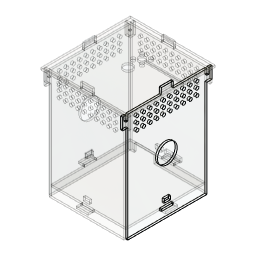
Cage_v8 (Autodesk Fusion 360 design; units mm, degrees)
Autodesk Fusion 360 part; units mm, degrees
(part 1 of 2)
sketch "Sketch1" plane through (0, 0, 0) normal (0, 0, 1) x (1, 0, 0)
  line L0 (-150, 3.175) -> (150, 3.175)
  line L1 (150, 3.175) -> (150, -3.175)
  line L2 (150, -3.175) -> (-150, -3.175)
  line L3 (-150, -3.175) -> (-150, 3.175)
  dimension "d1" = 300
  dimension "d2" = 150
  dimension "d3" = 6.35
  dimension "d4" = 3.175
  constraint horizontal L0
  constraint vertical L1
  constraint horizontal L2
  constraint vertical L3
  measures "d1" distance of L0.start L0.end
  measures "d2" distance of origin L3
  measures "d3" distance of L0.end L1.end
  measures "d4" distance of origin L0
extrude "Extrude1" add sketch "Sketch1" along normal blind 350 makes body 1
sketch "Sketch2" plane through (0, -3.175, 0) normal (0, -1, 0) x (1, 0, 0)
  line L0 (-150, 0) -> (150, 0)
  line L1 (150, 0) -> (150, 350)
  line L2 (150, 350) -> (-150, 350)
  line L3 (-150, 350) -> (-150, 0)
  line L4 (-120, 0) -> (120, 0)
  line L5 (120, 0) -> (120, 330.95)
  line L6 (120, 350) -> (-120, 350)
  line L7 (-120, 330.95) -> (-120, 0)
  line L8 (120, 350) -> (136.5, 350)
  line L9 (136.5, 350) -> (136.5, 311.9)
  line L10 (136.5, 311.9) -> (126.35, 311.9)
  line L11 (126.35, 311.9) -> (126.35, 330.95)
  line L12 (126.35, 330.95) -> (120, 330.95)
  line L13 (-120, 350) -> (-136.5, 350)
  line L14 (-136.5, 350) -> (-136.5, 311.9)
  line L15 (-136.5, 311.9) -> (-126.35, 311.9)
  line L16 (-126.35, 311.9) -> (-126.35, 330.95)
  line L17 (-126.35, 330.95) -> (-120, 330.95)
  dimension "d7" = 350
  dimension "d8" = 240
  dimension "d9" = 120
  dimension "d10" = 6.35
  dimension "d14" = 38.1
  dimension "d15" = 19.05
  dimension "d18" = 6.35
  dimension "d20" = 273
  dimension "d21" = 38.1
  dimension "d22" = 19.05
  constraint horizontal L4
  constraint vertical L5
  constraint horizontal L6
  constraint vertical L7
  constraint coincident L0 L4.start
  constraint coincident L2 L8.end
  constraint perpendicular L5 L8
  constraint perpendicular L2 L9
  constraint perpendicular L9 L10
  constraint perpendicular L10 L11
  constraint perpendicular L5 L12
  constraint coincident L2 L13.end
  constraint perpendicular L7 L13
  constraint perpendicular L13 L14
  constraint perpendicular L14 L15
  constraint perpendicular L15 L16
  constraint perpendicular L7 L17
  constraint equal L10 L15
  measures "d7" distance of L4.end L6.start
  measures "d8" distance of L4.start L4.end
  measures "d9" distance of origin L7
  measures "d10" distance of L11.end L5.end
  measures "d14" distance of L8.end L9.end
  measures "d15" distance of L8 L12
  measures "d18" distance of L16.end L7.start
  measures "d20" distance of L9 L14
  measures "d21" distance of L13.end L14.end
  measures "d22" distance of L13 L17
extrude "Extrude2" cut sketch "Sketch2" against normal blind 140 contours L0 L2 L3 L7 L14 L15 L16 L17 | L0 L1 L2 L5 L9 L10 L11 L12 bodies 1
sketch "Sketch3" plane through (0, 0, 350) normal (0, 0, 1) x (-1, 0, 0)
  line L0 (136.5, -3.175) -> (136.5, 3.175)
  line L1 (136.5, 3.175) -> (-136.5, 3.175)
  line L2 (-136.5, 3.175) -> (-136.5, -3.175)
  line L3 (-136.5, -3.175) -> (136.5, -3.175)
  line L4 (19.05, -3.175) -> (-19.05, -3.175)
  line L5 (-19.05, -3.175) -> (-19.05, 3.175)
  line L6 (-19.05, 3.175) -> (19.05, 3.175)
  line L7 (19.05, 3.175) -> (19.05, -3.175)
  dimension "d25" = 38.1
  dimension "d26" = 19.05
  constraint horizontal L4
  constraint vertical L5
  constraint horizontal L6
  constraint vertical L7
  constraint coincident L1 L5.end
  constraint coincident L3 L4.start
  measures "d25" distance of L4.start L4.end
  measures "d26" distance of origin L7
extrude "Extrude3" add sketch "Sketch3" along normal blind 20 contours L1 L3 L4 L5 L6 L7 bodies 1
sketch "Sketch4" plane through (0, -3.175, 0) normal (0, -1, 0) x (1, 0, 0)
  line L0 (-136.5, 350) -> (-136.5, 311.9)
  line L1 (-136.5, 311.9) -> (-126.35, 311.9)
  line L2 (-126.35, 311.9) -> (-126.35, 330.95)
  line L3 (-126.35, 330.95) -> (-120, 330.95)
  line L4 (-120, 330.95) -> (-120, 0)
  line L5 (-120, 0) -> (120, 0)
  line L6 (120, 0) -> (120, 330.95)
  line L7 (120, 330.95) -> (126.35, 330.95)
  line L8 (126.35, 330.95) -> (126.35, 311.9)
  line L9 (126.35, 311.9) -> (136.5, 311.9)
  line L10 (136.5, 311.9) -> (136.5, 350)
  line L11 (136.5, 350) -> (19.05, 350)
  line L12 (19.05, 350) -> (19.05, 370)
  line L13 (19.05, 370) -> (-19.05, 370)
  line L14 (-19.05, 370) -> (-19.05, 350)
  line L15 (-19.05, 350) -> (-136.5, 350)
  circle A0 centre (-90, 330) radius 5
  circle A1 centre (-70, 330) radius 5
  circle A2 centre (-50, 330) radius 5
  circle A3 centre (-30, 330) radius 5
  circle A4 centre (-10, 330) radius 5
  circle A5 centre (10, 330) radius 5
  circle A6 centre (30, 330) radius 5
  circle A7 centre (50, 330) radius 5
  circle A8 centre (70, 330) radius 5
  circle A9 centre (90, 330) radius 5
  circle A10 centre (-90, 310) radius 5
  circle A11 centre (-70, 310) radius 5
  circle A12 centre (-50, 310) radius 5
  circle A13 centre (-30, 310) radius 5
  circle A14 centre (-10, 310) radius 5
  circle A15 centre (10, 310) radius 5
  circle A16 centre (30, 310) radius 5
  circle A17 centre (50, 310) radius 5
  circle A18 centre (70, 310) radius 5
  circle A19 centre (90, 310) radius 5
  circle A20 centre (-90, 290) radius 5
  circle A21 centre (-70, 290) radius 5
  circle A22 centre (-50, 290) radius 5
  circle A23 centre (-30, 290) radius 5
  circle A24 centre (-10, 290) radius 5
  circle A25 centre (10, 290) radius 5
  circle A26 centre (30, 290) radius 5
  circle A27 centre (50, 290) radius 5
  circle A28 centre (70, 290) radius 5
  circle A29 centre (90, 290) radius 5
  dimension "d29" = 30
  dimension "d30" = 20
  dimension "d31" = 10
  dimension "d32" = 10
  dimension "d33" = 20
  dimension "d34" = 20
  dimension "d35" = 20
  dimension "d36" = 20
  dimension "d37" = 20
  dimension "d38" = 20
  dimension "d39" = 20
  dimension "d40" = 20
  dimension "d41" = 30
  dimension "d42" = 30
  dimension "d52" = 10
  dimension "d53" = 20
  dimension "d54" = 20
  dimension "d55" = 20
  dimension "d56" = 20
  dimension "d57" = 20
  dimension "d58" = 20
  dimension "d59" = 20
  dimension "d60" = 20
  dimension "d61" = 20
  dimension "d62" = 10
  dimension "d63" = 10
  constraint equal A7 A9
  constraint equal A6 A9
  constraint equal A5 A9
  constraint equal A4 A8
  constraint equal A3 A8
  constraint equal A2 A8
  constraint equal A1 A9
  constraint equal A0 A8
  constraint equal A18 A19
  constraint equal A17 A19
  constraint equal A16 A19
  constraint equal A15 A19
  constraint equal A14 A19
  constraint equal A13 A19
  constraint equal A12 A19
  constraint equal A11 A19
  constraint equal A10 A19
  measures "d29" distance of L6 A9.centre
  measures "d30" distance of A8.centre A9.centre
  measures "d31" diameter of A9
  measures "d32" diameter of A8
  measures "d33" distance of A7.centre A8.centre
  measures "d34" distance of A6.centre A7.centre
  measures "d35" distance of A5.centre A6.centre
  measures "d36" distance of A4.centre A5.centre
  measures "d37" distance of A3.centre A4.centre
  measures "d38" distance of A2.centre A3.centre
  measures "d39" distance of A1.centre A2.centre
  measures "d40" distance of A0.centre A1.centre
  measures "d41" distance of L4 A10.centre
  measures "d42" distance of L6 A19.centre
  measures "d52" diameter of A19
  measures "d53" distance of A18.centre A19.centre
  measures "d54" distance of A17.centre A18.centre
  measures "d55" distance of A16.centre A17.centre
  measures "d56" distance of A15.centre A16.centre
  measures "d57" distance of A14.centre A15.centre
  measures "d58" distance of A13.centre A14.centre
  measures "d59" distance of A12.centre A13.centre
  measures "d60" distance of A11.centre A12.centre
  measures "d61" distance of A10.centre A11.centre
  measures "d62" diameter of A20
  measures "d63" diameter of A21
extrude "Extrude4" cut sketch "Sketch4" against normal blind 35 contours A0 | A1 | A2 | A3 | A4 | A5 | A6 | A7 | A8 | A9 | A10 | A11 | A12 | A13 | A14 | A15 | A16 | A17 | A18 | A19 | A20 | A21 | A22 | A23 | A24 | A25 | A26 | A27 | A28 | A29 bodies 1
ref_plane "WorkPlane1" through (120, 0, 0) normal (1, 0, 0) x (0, 1, 0) in component "Right wall"
sketch "Sketch1 (2)" plane through (120, 0, 0) normal (1, 0, 0) x (0, 1, 0) in component "Right wall"
  line L0 (3.175, 0) -> (257.175, 0)
  line L1 (257.175, 0) -> (257.175, 350)
  line L2 (257.175, 350) -> (3.175, 350)
  line L3 (3.175, 350) -> (3.175, 0)
  dimension "d67" = 3.175
  dimension "d68" = 254
  dimension "d69" = 350
  constraint horizontal L0
  constraint vertical L1
  constraint horizontal L2
  constraint vertical L3
  measures "d67" distance of origin L0.start
  measures "d68" distance of L0.start L0.end
  measures "d69" distance of L0.end L1.end
extrude "Extrude1'" add sketch "Sketch1 (2)" along normal blind 6.35 separate body makes body 2 in component "Right wall"
sketch "Sketch2 (2)" plane through (0, 0, 350) normal (0, 0, 1) x (-1, 0, 0) in component "Right wall"
  line L0 (-120, -257.175) -> (-120, -3.175)
  line L1 (-120, -3.175) -> (-126.35, -3.175)
  line L2 (-126.35, -3.175) -> (-126.35, -257.175)
  line L3 (-126.35, -257.175) -> (-120, -257.175)
  line L4 (-126.35, -111.125) -> (-120, -111.125)
  line L5 (-120, -111.125) -> (-120, -149.225)
  line L6 (-120, -149.225) -> (-126.35, -149.225)
  line L7 (-126.35, -149.225) -> (-126.35, -111.125)
  dimension "d72" = 38.1
  dimension "d73" = 107.95
  constraint horizontal L4
  constraint vertical L5
  constraint horizontal L6
  constraint vertical L7
  constraint coincident L0 L5.end
  constraint coincident L2 L4.start
  measures "d72" distance of L4.end L5.end
  measures "d73" distance of L1 L4
extrude "Extrude2'" add sketch "Sketch2 (2)" along normal blind 20 contours L0 L2 L4 L5 L6 L7 bodies 2 in component "Right wall"
sketch "Sketch3 (2)" plane through (126.35, 0, 0) normal (1, 0, 0) x (0, 1, 0) in component "Right wall"
  line L0 (3.175, 350) -> (3.175, 0)
  line L1 (3.175, 0) -> (257.175, 0)
  line L2 (257.175, 0) -> (257.175, 350)
  line L3 (257.175, 350) -> (149.225, 350)
  line L4 (149.225, 350) -> (149.225, 370)
  line L5 (149.225, 370) -> (111.125, 370)
  line L6 (111.125, 370) -> (111.125, 350)
  line L7 (111.125, 350) -> (3.175, 350)
  circle A0 centre (33.875, 330) radius 5
  circle A1 centre (55.275, 330) radius 5
  circle A2 centre (76.675, 330) radius 5
  circle A3 centre (98.075, 330) radius 5
  circle A4 centre (119.475, 330) radius 5
  circle A5 centre (140.875, 330) radius 5
  circle A6 centre (162.275, 330) radius 5
  circle A7 centre (183.675, 330) radius 5
  circle A8 centre (205.075, 330) radius 5
  circle A9 centre (226.475, 330) radius 5
  circle A10 centre (33.875, 310) radius 5
  circle A11 centre (55.275, 310) radius 5
  circle A12 centre (76.675, 310) radius 5
  circle A13 centre (98.075, 310) radius 5
  circle A14 centre (119.475, 310) radius 5
  circle A15 centre (140.875, 310) radius 5
  circle A16 centre (162.275, 310) radius 5
  circle A17 centre (183.675, 310) radius 5
  circle A18 centre (205.075, 310) radius 5
  circle A19 centre (226.4722, 310.344) radius 5
  circle A20 centre (33.875, 290) radius 5
  circle A21 centre (55.275, 290) radius 5
  circle A22 centre (119.475, 290) radius 5
  circle A23 centre (140.875, 290) radius 5
  circle A24 centre (162.275, 290) radius 5
  circle A25 centre (98.075, 290) radius 5
  circle A26 centre (76.675, 290) radius 5
  circle A27 centre (183.675, 290) radius 5
  circle A28 centre (205.075, 290) radius 5
  circle A29 centre (226.475, 290) radius 5
  dimension "d76" = 20
  dimension "d77" = 10
  dimension "d78" = 30.7
  dimension "d79" = 21.4
  dimension "d80" = 21.4
  dimension "d81" = 21.4
  dimension "d82" = 21.4
  dimension "d85" = 21.4
  dimension "d86" = 21.4
  dimension "d87" = 21.4
  dimension "d88" = 21.4
  dimension "d90" = 20
  dimension "d91" = 10
  dimension "d92" = 30.7
  dimension "d93" = 21.4
  dimension "d94" = 21.4
  dimension "d95" = 21.4
  dimension "d96" = 21.4
  dimension "d99" = 21.4
  dimension "d100" = 21.4
  dimension "d101" = 21.4
  dimension "d102" = 21.4
  dimension "d103" = 21.4
  dimension "d104" = 21.4
  dimension "d105" = 10
  dimension "d106" = 21.4
  dimension "d107" = 21.4
  dimension "d108" = 21.4
  dimension "d109" = 21.4
  dimension "d110" = 21.4
  dimension "d111" = 21.4
  dimension "d112" = 21.4
  dimension "d113" = 21.4
  dimension "d114" = 21.4
  dimension "d211" = 20
  dimension "d212" = 30.7
  constraint equal A0 A1
  constraint equal A0 A2
  constraint equal A0 A3
  constraint equal A3 A4
  constraint equal A5 A6
  constraint equal A6 A7
  constraint equal A7 A8
  constraint equal A8 A9
  constraint collinear A0.centre A1.centre A2.centre
  constraint collinear A5.centre A6.centre A7.centre
  constraint collinear A7.centre A8.centre A9.centre
  constraint collinear A10.centre A11.centre A12.centre
  constraint equal A10 A11
  constraint equal A11 A12
  constraint equal A12 A13
  constraint equal A13 A14
  constraint equal A15 A16
  constraint equal A16 A17
  constraint equal A17 A18
  constraint equal A18 A19
  constraint equal A14 A15
  constraint equal A4 A5
  constraint collinear A26.centre A20.centre A21.centre
  constraint equal A20 A21
  constraint equal A21 A26
  constraint equal A25 A26
  constraint equal A22 A25
  constraint equal A23 A24
  constraint equal A24 A27
  constraint equal A27 A28
  constraint equal A28 A29
  constraint equal A22 A23
  measures "d76" distance of L7 A0.centre
  measures "d77" diameter of A0
  measures "d78" distance of L0 A0.centre
  measures "d79" distance of A0.centre A1.centre
  measures "d80" distance of A1.centre A2.centre
  measures "d81" distance of A2.centre A3.centre
  measures "d82" distance of A3.centre A4.centre
  measures "d85" distance of A5.centre A6.centre
  measures "d86" distance of A6.centre A7.centre
  measures "d87" distance of A7.centre A8.centre
  measures "d88" distance of A8.centre A9.centre
  measures "d90" vertical distance of A0.centre A10.centre
  measures "d91" diameter of A10
  measures "d92" distance of L0 A10.centre
  measures "d93" distance of A10.centre A11.centre
  measures "d94" distance of A11.centre A12.centre
  measures "d95" distance of A12.centre A13.centre
  measures "d96" distance of A13.centre A14.centre
  measures "d99" distance of A15.centre A16.centre
  measures "d100" distance of A16.centre A17.centre
  measures "d101" distance of A17.centre A18.centre
  measures "d102" distance of A18.centre A19.centre
  measures "d103" distance of A4.centre A5.centre
  measures "d104" distance of A14.centre A15.centre
  measures "d105" diameter of A20
  measures "d106" distance of A20.centre A21.centre
  measures "d107" distance of A26.centre A21.centre
  measures "d108" distance of A26.centre A25.centre
  measures "d109" distance of A25.centre A22.centre
  measures "d110" distance of A23.centre A24.centre
  measures "d111" distance of A27.centre A24.centre
  measures "d112" distance of A27.centre A28.centre
  measures "d113" distance of A29.centre A28.centre
  measures "d114" distance of A23.centre A22.centre
  measures "d211" vertical distance of A10.centre A20.centre
  measures "d212" distance of L2 A29.centre
extrude "Extrude3'" cut sketch "Sketch3 (2)" against normal blind 40 contours A0 | A1 | A2 | A3 | A4 | A5 | A6 | A7 | A8 | A9 | A10 | A11 | A12 | A13 | A14 | A15 | A16 | A17 | A18 | A19 | A20 | A21 | A22 | A23 | A24 | A25 | A26 | A27 | A28 | A29 bodies 2 in component "Right wall"
sketch "Sketch5" plane through (126.35, 0, 0) normal (1, 0, 0) x (0, 1, 0) in component "Right wall"
  circle A0 centre (183.675, 290) radius 5
  circle A1 centre (98.075, 290) radius 5
  circle A2 centre (33.875, 310) radius 5
  circle A3 centre (119.475, 310) radius 5
  circle A4 centre (205.075, 310) radius 5
  circle A5 centre (183.675, 330) radius 5
  circle A6 centre (98.075, 330) radius 5
  circle A7 centre (33.875, 330) radius 5
  circle A8 centre (119.475, 330) radius 5
  circle A9 centre (205.075, 330) radius 5
  circle A10 centre (183.675, 310) radius 5
  circle A11 centre (98.075, 310) radius 5
  circle A12 centre (33.875, 290) radius 5
  circle A13 centre (119.475, 290) radius 5
  circle A14 centre (205.075, 290) radius 5
  circle A15 centre (162.275, 290) radius 5
  circle A16 centre (76.675, 290) radius 5
  circle A17 centre (55.275, 310) radius 5
  circle A18 centre (162.275, 310) radius 5
  circle A19 centre (226.4722, 310.344) radius 5
  circle A20 centre (162.275, 330) radius 5
  circle A21 centre (76.675, 330) radius 5
  circle A22 centre (55.275, 330) radius 5
  circle A23 centre (140.875, 330) radius 5
  circle A24 centre (226.475, 330) radius 5
  circle A25 centre (140.875, 310) radius 5
  circle A26 centre (76.675, 310) radius 5
  circle A27 centre (55.275, 290) radius 5
  circle A28 centre (140.875, 290) radius 5
  circle A29 centre (226.475, 290) radius 5
  line L0 (3.175, 350) -> (3.175, 0)
  line L1 (3.175, 0) -> (257.175, 0)
  line L2 (257.175, 0) -> (257.175, 350)
  line L3 (257.175, 350) -> (149.225, 350)
  line L4 (149.225, 350) -> (149.225, 370)
  line L5 (149.225, 370) -> (111.125, 370)
  line L6 (111.125, 370) -> (111.125, 350)
  line L7 (111.125, 350) -> (3.175, 350)
  line L8 (3.175, 311.9) -> (-13.325, 311.9)
  line L9 (-3.175, 330.95) -> (3.175, 330.95)
  line L10 (3.175, 330.95) -> (3.175, 311.9)
  line L11 (-13.325, 350) -> (-3.175, 350)
  line L12 (-3.175, 350) -> (-3.175, 330.95)
  line L13 (257.175, 311.9) -> (273.675, 311.9)
  line L14 (273.675, 311.9) -> (273.675, 350)
  line L15 (273.675, 350) -> (263.525, 350)
  line L16 (263.525, 350) -> (263.525, 330.95)
  line L17 (263.525, 330.95) -> (257.175, 330.95)
  line L18 (-13.325, 350) -> (-13.325, 311.9)
  dimension "d119" = 19.05
  dimension "d124" = 6.35
  dimension "d127" = 6.35
  dimension "d128" = 10.15
  dimension "d130" = 19.05
  dimension "d131" = 19.05
  dimension "d132" = 19.05
  dimension "d133" = 19.05
  constraint horizontal L8
  constraint horizontal L9
  constraint vertical L10
  constraint coincident L0 L8.start
  constraint horizontal L11
  constraint vertical L12
  constraint coincident L2 L13.start
  constraint perpendicular L2 L13
  constraint perpendicular L13 L14
  constraint perpendicular L14 L15
  constraint perpendicular L15 L16
  constraint coincident L2 L17.end
  constraint perpendicular L2 L17
  constraint perpendicular L8 L18
  measures "d119" distance of L7 L9
  measures "d124" distance of L0 L12
  measures "d127" distance of L16.end L17.end
  measures "d128" distance of L14.end L15.end
  measures "d130" distance of L13 L17
  measures "d131" distance of L15.end L16.end
  measures "d132" distance of L9 L11
  measures "d133" distance of L8 L9
extrude "Extrude4'" add sketch "Sketch5" against normal blind 6.35 contours L0 L8 L9 L10 L11 L12 L18 | L2 L13 L14 L15 L16 L17 bodies 2 in component "Right wall"
sketch "Sketch5 (2)" plane through (0, -3.175, 0) normal (0, -1, 0) x (1, 0, 0)
  circle A0 centre (50, 290) radius 5
  circle A1 centre (-30, 290) radius 5
  circle A2 centre (-90, 310) radius 5
  circle A3 centre (-10, 310) radius 5
  circle A4 centre (70, 310) radius 5
  circle A5 centre (50, 330) radius 5
  circle A6 centre (-30, 330) radius 5
  circle A7 centre (-90, 330) radius 5
  circle A8 centre (-10, 330) radius 5
  circle A9 centre (70, 330) radius 5
  circle A10 centre (50, 310) radius 5
  circle A11 centre (-30, 310) radius 5
  circle A12 centre (-90, 290) radius 5
  circle A13 centre (-10, 290) radius 5
  circle A14 centre (70, 290) radius 5
  circle A15 centre (30, 290) radius 5
  circle A16 centre (-50, 290) radius 5
  circle A17 centre (-70, 310) radius 5
  circle A18 centre (10, 310) radius 5
  circle A19 centre (90, 310) radius 5
  circle A20 centre (30, 330) radius 5
  circle A21 centre (-50, 330) radius 5
  circle A22 centre (-70, 330) radius 5
  circle A23 centre (10, 330) radius 5
  circle A24 centre (90, 330) radius 5
  circle A25 centre (30, 310) radius 5
  circle A26 centre (-50, 310) radius 5
  circle A27 centre (-70, 290) radius 5
  circle A28 centre (10, 290) radius 5
  circle A29 centre (90, 290) radius 5
  line L0 (-136.5, 350) -> (-136.5, 311.9)
  line L1 (-136.5, 311.9) -> (-126.35, 311.9)
  line L2 (-126.35, 311.9) -> (-126.35, 330.95)
  line L3 (-126.35, 330.95) -> (-120, 330.95)
  line L4 (-120, 330.95) -> (-120, 0)
  line L5 (-120, 0) -> (120, 0)
  line L6 (120, 0) -> (120, 330.95)
  line L7 (120, 330.95) -> (126.35, 330.95)
  line L8 (126.35, 330.95) -> (126.35, 311.9)
  line L9 (126.35, 311.9) -> (136.5, 311.9)
  line L10 (136.5, 311.9) -> (136.5, 350)
  line L11 (136.5, 350) -> (19.05, 350)
  line L12 (19.05, 350) -> (19.05, 370)
  line L13 (19.05, 370) -> (-19.05, 370)
  line L14 (-19.05, 370) -> (-19.05, 350)
  line L15 (-19.05, 350) -> (-136.5, 350)
  line L16 (-19.05, 31.75) -> (19.05, 31.75)
  line L17 (19.05, 31.75) -> (19.05, 25.4)
  line L18 (19.05, 25.4) -> (-19.05, 25.4)
  line L19 (-19.05, 25.4) -> (-19.05, 31.75)
  dimension "d136" = 38.1
  dimension "d137" = 19.05
  dimension "d138" = 6.35
  dimension "d139" = 25.4
  constraint horizontal L16
  constraint vertical L17
  constraint horizontal L18
  constraint vertical L19
  measures "d136" distance of L16.start L16.end
  measures "d137" distance of origin L19
  measures "d138" distance of L16.end L17.end
  measures "d139" distance of L5 L18
extrude "Extrude5" cut sketch "Sketch5 (2)" against normal blind 6.35 contours L16 L17 L18 L19 bodies 1
sketch "Sketch6" plane through (126.35, 0, 0) normal (1, 0, 0) x (0, 1, 0) in component "Right wall"
  circle A0 centre (183.675, 290) radius 5
  circle A1 centre (98.075, 290) radius 5
  circle A2 centre (33.875, 310) radius 5
  circle A3 centre (119.475, 310) radius 5
  circle A4 centre (205.075, 310) radius 5
  circle A5 centre (183.675, 330) radius 5
  circle A6 centre (98.075, 330) radius 5
  circle A7 centre (33.875, 330) radius 5
  circle A8 centre (119.475, 330) radius 5
  circle A9 centre (205.075, 330) radius 5
  circle A10 centre (183.675, 310) radius 5
  circle A11 centre (98.075, 310) radius 5
  circle A12 centre (33.875, 290) radius 5
  circle A13 centre (119.475, 290) radius 5
  circle A14 centre (205.075, 290) radius 5
  circle A15 centre (162.275, 290) radius 5
  circle A16 centre (76.675, 290) radius 5
  circle A17 centre (55.275, 310) radius 5
  circle A18 centre (162.275, 310) radius 5
  circle A19 centre (226.4722, 310.344) radius 5
  circle A20 centre (162.275, 330) radius 5
  circle A21 centre (76.675, 330) radius 5
  circle A22 centre (55.275, 330) radius 5
  circle A23 centre (140.875, 330) radius 5
  circle A24 centre (226.475, 330) radius 5
  circle A25 centre (140.875, 310) radius 5
  circle A26 centre (76.675, 310) radius 5
  circle A27 centre (55.275, 290) radius 5
  circle A28 centre (140.875, 290) radius 5
  circle A29 centre (226.475, 290) radius 5
  line L0 (3.175, 350) -> (3.175, 330.95)
  line L1 (3.175, 330.95) -> (-3.175, 330.95)
  line L2 (-3.175, 330.95) -> (-3.175, 350)
  line L3 (-3.175, 350) -> (-13.325, 350)
  line L4 (-13.325, 350) -> (-13.325, 311.9)
  line L5 (-13.325, 311.9) -> (3.175, 311.9)
  line L6 (3.175, 311.9) -> (3.175, 0)
  line L7 (3.175, 0) -> (257.175, 0)
  line L8 (257.175, 0) -> (257.175, 311.9)
  line L9 (257.175, 311.9) -> (273.675, 311.9)
  line L10 (273.675, 311.9) -> (273.675, 350)
  line L11 (273.675, 350) -> (263.525, 350)
  line L12 (263.525, 350) -> (263.525, 330.95)
  line L13 (263.525, 330.95) -> (257.175, 330.95)
  line L14 (257.175, 330.95) -> (257.175, 350)
  line L15 (257.175, 350) -> (149.225, 350)
  line L16 (149.225, 350) -> (149.225, 370)
  line L17 (149.225, 370) -> (111.125, 370)
  line L18 (111.125, 370) -> (111.125, 350)
  line L19 (111.125, 350) -> (3.175, 350)
  line L20 (111.125, 31.75) -> (149.225, 31.75)
  line L21 (149.225, 31.75) -> (149.225, 25.4)
  line L22 (149.225, 25.4) -> (111.125, 25.4)
  line L23 (111.125, 25.4) -> (111.125, 31.75)
  dimension "d142" = 38.1
  dimension "d143" = 6.35
  dimension "d144" = 25.4
  dimension "d145" = 107.95
  constraint horizontal L20
  constraint vertical L21
  constraint horizontal L22
  constraint vertical L23
  measures "d142" distance of L20.start L20.end
  measures "d143" distance of L20.start L22.end
  measures "d144" distance of L7 L22
  measures "d145" distance of L6 L23
extrude "Extrude5'" cut sketch "Sketch6" against normal blind 20 contours L20 L21 L22 L23 bodies 2 in component "Right wall"
copy_body "CopyPasteBodies1" bodies 2 makes body 3
move_body "Move1" bodies 3 to x (1, 0, 0) y (0, 1, 0) z (0, 0, 1) at (-246.35, 0, 0)
copy_body "CopyPasteBodies2" bodies 1 makes body 4
move_body "Move2" bodies 4 to x (1, 0, 0) y (0, 1, 0) z (0, 0, 1) at (0, 260.35, 0)
copy_body "Body->Comp1" bodies 4 removing the originals makes body 5 in component "Back Wall"
copy_body "Body->Comp2" bodies 3 removing the originals makes body 6 in component "Left Wall"
copy_body "Body->Comp3" bodies 1 removing the originals makes body 7 in component "Front Wall"
ref_plane "WorkPlane1" through (0, 0, 25.4) normal (0, 0, 1) x (1, 0, 0) in component "Floor"
sketch "Sketch1 (3)" plane through (0, 0, 25.4) normal (0, 0, 1) x (1, 0, 0) in component "Floor"
  line L0 (-120, 3.175) -> (120, 3.175)
  line L1 (120, 3.175) -> (120, 257.175)
  line L2 (120, 257.175) -> (-120, 257.175)
  line L3 (-120, 257.175) -> (-120, 3.175)
  dimension "d153" = 240
  dimension "d154" = 254
  dimension "d155" = 120
  dimension "d156" = 3.175
  constraint horizontal L0
  constraint vertical L1
  constraint horizontal L2
  constraint vertical L3
  measures "d153" distance of L1.end L2.end
  measures "d154" distance of L0.end L1.end
  measures "d155" distance of origin L3
  measures "d156" distance of origin L0
extrude "Extrude1''" add sketch "Sketch1 (3)" along normal blind 6.35 separate body makes body 8 in component "Floor"
sketch "Sketch2 (3)" plane through (-120, 0, 0) normal (-1, 0, 0) x (0, -1, 0) in component "Floor"
  line L0 (-257.175, 25.4) -> (-3.175, 25.4)
  line L1 (-3.175, 25.4) -> (-3.175, 31.75)
  line L2 (-3.175, 31.75) -> (-257.175, 31.75)
  line L3 (-257.175, 31.75) -> (-257.175, 25.4)
  line L4 (-149.225, 31.75) -> (-111.125, 31.75)
  line L5 (-111.125, 31.75) -> (-111.125, 25.4)
  line L6 (-111.125, 25.4) -> (-149.225, 25.4)
  line L7 (-149.225, 25.4) -> (-149.225, 31.75)
  dimension "d159" = 38.1
  dimension "d160" = 107.95
  constraint horizontal L4
  constraint vertical L5
  constraint horizontal L6
  constraint vertical L7
  constraint coincident L0 L5.end
  constraint coincident L2 L4.start
  measures "d159" distance of L4.start L4.end
  measures "d160" distance of L1 L5
extrude "Extrude2''" add sketch "Sketch2 (3)" along normal blind 20 contours L0 L2 L4 L5 L6 L7 bodies 8 in component "Floor"
sketch "Sketch3 (3)" plane through (0, 257.175, 0) normal (0, 1, 0) x (-1, 0, 0) in component "Floor"
  line L0 (-120, 25.4) -> (120, 25.4)
  line L1 (120, 25.4) -> (120, 31.75)
  line L2 (120, 31.75) -> (-120, 31.75)
  line L3 (-120, 31.75) -> (-120, 25.4)
  line L4 (-19.05, 31.75) -> (19.05, 31.75)
  line L5 (19.05, 31.75) -> (19.05, 25.4)
  line L6 (19.05, 25.4) -> (-19.05, 25.4)
  line L7 (-19.05, 25.4) -> (-19.05, 31.75)
  dimension "d163" = 38.1
  dimension "d164" = 100.95
  constraint horizontal L4
  constraint vertical L5
  constraint horizontal L6
  constraint vertical L7
  constraint coincident L0 L5.end
  constraint coincident L2 L4.start
  measures "d163" distance of L4.start L4.end
  measures "d164" distance of L1 L5
extrude "Extrude3''" add sketch "Sketch3 (3)" along normal blind 20 contours L0 L2 L4 L5 L6 L7 bodies 8 in component "Floor"
sketch "Sketch4 (2)" plane through (120, 0, 0) normal (1, 0, 0) x (0, 1, 0) in component "Floor"
  line L0 (3.175, 25.4) -> (257.175, 25.4)
  line L1 (257.175, 25.4) -> (257.175, 31.75)
  line L2 (257.175, 31.75) -> (3.175, 31.75)
  line L3 (3.175, 31.75) -> (3.175, 25.4)
  line L4 (111.125, 31.75) -> (149.225, 31.75)
  line L5 (149.225, 31.75) -> (149.225, 25.4)
  line L6 (149.225, 25.4) -> (111.125, 25.4)
  line L7 (111.125, 25.4) -> (111.125, 31.75)
  dimension "d167" = 38.1
  dimension "d168" = 107.95
  constraint horizontal L4
  constraint vertical L5
  constraint horizontal L6
  constraint vertical L7
  constraint coincident L0 L5.end
  constraint coincident L2 L4.start
  measures "d167" distance of L4.start L4.end
  measures "d168" distance of L3 L7
extrude "Extrude4''" add sketch "Sketch4 (2)" along normal blind 20 contours L0 L2 L4 L5 L6 L7 bodies 8 in component "Floor"
sketch "Sketch5 (3)" plane through (0, 3.175, 0) normal (0, -1, 0) x (1, 0, 0) in component "Floor"
  line L0 (-120, 25.4) -> (120, 25.4)
  line L1 (120, 25.4) -> (120, 31.75)
  line L2 (120, 31.75) -> (-120, 31.75)
  line L3 (-120, 31.75) -> (-120, 25.4)
  line L4 (-19.05, 31.75) -> (19.05, 31.75)
  line L5 (19.05, 31.75) -> (19.05, 25.4)
  line L6 (19.05, 25.4) -> (-19.05, 25.4)
  line L7 (-19.05, 25.4) -> (-19.05, 31.75)
  dimension "d171" = 38.1
  dimension "d172" = 100.95
  constraint horizontal L4
  constraint vertical L5
  constraint horizontal L6
  constraint vertical L7
  constraint coincident L0 L5.end
  constraint coincident L2 L4.start
  measures "d171" distance of L4.start L4.end
  measures "d172" distance of L3 L7
extrude "Extrude5''" add sketch "Sketch5 (3)" along normal blind 20 contours L0 L2 L4 L5 L6 L7 bodies 8 in component "Floor"
ref_plane "WorkPlane1" through (0, 0, 350) normal (0, 0, 1) x (1, 0, 0) in component "Roof"
sketch "Sketch1 (4)" plane through (0, 0, 350) normal (0, 0, 1) x (1, 0, 0) in component "Roof"
  line L0 (-136.35, 273.775) -> (136.35, 273.775)
  line L1 (136.35, 273.775) -> (136.35, -13.325)
  line L2 (136.35, -13.325) -> (-136.35, -13.325)
  line L3 (-136.35, -13.325) -> (-136.35, 273.775)
  line L4 (-19.05, 257.175) -> (19.05, 257.175)
  line L5 (19.05, 257.175) -> (19.05, 263.525)
  line L6 (19.05, 263.525) -> (-19.05, 263.525)
  line L7 (-19.05, 263.525) -> (-19.05, 257.175)
  line L8 (120, 149.225) -> (126.35, 149.225)
  line L9 (126.35, 149.225) -> (126.35, 111.125)
  line L10 (126.35, 111.125) -> (120, 111.125)
  line L11 (120, 111.125) -> (120, 149.225)
  line L12 (-19.05, 3.275) -> (19.05, 3.275)
  line L13 (19.05, 3.275) -> (19.05, -3.075)
  line L14 (19.05, -3.075) -> (-19.05, -3.075)
  line L15 (-19.05, -3.075) -> (-19.05, 3.275)
  line L16 (-126.35, 149.2333) -> (-120, 149.2333)
  line L17 (-120, 149.2333) -> (-120, 111.1333)
  line L18 (-120, 111.1333) -> (-126.35, 111.1333)
  line L19 (-126.35, 111.1333) -> (-126.35, 149.2333)
  dimension "d176" = 287.1
  dimension "d177" = 13.325
  dimension "d178" = 272.7
  dimension "d179" = 136.35
  dimension "d180" = 6.35
  dimension "d181" = 38.1
  dimension "d182" = 19.05
  dimension "d183" = 10.25
  dimension "d184" = 38.1
  dimension "d185" = 6.35
  dimension "d186" = 10
  dimension "d187" = 124.55
  dimension "d188" = 38.1
  dimension "d189" = 6.35
  dimension "d190" = 38.1
  dimension "d191" = 6.35
  dimension "d193" = 19.05
  dimension "d194" = 3.275
  constraint horizontal L0
  constraint vertical L1
  constraint horizontal L2
  constraint vertical L3
  constraint horizontal L4
  constraint vertical L5
  constraint horizontal L6
  constraint vertical L7
  constraint horizontal L8
  constraint vertical L9
  constraint horizontal L10
  constraint vertical L11
  constraint horizontal L12
  constraint vertical L13
  constraint horizontal L14
  constraint vertical L15
  constraint horizontal L16
  constraint vertical L17
  constraint horizontal L18
  constraint vertical L19
  measures "d176" distance of L0.start L2.end
  measures "d177" distance of origin L2
  measures "d178" distance of L1.end L2.end
  measures "d179" distance of origin L3
  measures "d180" distance of L4.start L6.end
  measures "d181" distance of L4.start L4.end
  measures "d182" distance of origin L7
  measures "d183" distance of L0 L6
  measures "d184" distance of L8.start L10.end
  measures "d185" distance of L8.start L8.end
  measures "d186" distance of L1 L9
  measures "d187" distance of L0 L8.end
  measures "d188" distance of L16.end L17.end
  measures "d189" distance of L17.end L18.end
  measures "d190" distance of L12.start L12.end
  measures "d191" distance of L12.end L13.end
  measures "d193" distance of origin L15
  measures "d194" distance of origin L12
extrude "Extrude1'''" add sketch "Sketch1 (4)" along normal blind 6.35 separate body makes body 9 in component "Roof"
sketch "Sketch1 (5)" plane through (0, 263.525, 0) normal (0, 1, 0) x (-1, 0, 0) in component "Back Wall"
  line L0 (-19.05, 25.4) -> (-19.05, 31.75)
  line L1 (-19.05, 31.75) -> (19.05, 31.75)
  line L2 (19.05, 31.75) -> (19.05, 25.4)
  line L3 (19.05, 25.4) -> (-19.05, 25.4)
  circle A0 centre (-50, 290) radius 5
  circle A1 centre (30, 290) radius 5
  circle A2 centre (90, 310) radius 5
  circle A3 centre (10, 310) radius 5
  circle A4 centre (-70, 310) radius 5
  circle A5 centre (-50, 330) radius 5
  circle A6 centre (30, 330) radius 5
  circle A7 centre (90, 330) radius 5
  circle A8 centre (10, 330) radius 5
  circle A9 centre (-70, 330) radius 5
  circle A10 centre (-50, 310) radius 5
  circle A11 centre (30, 310) radius 5
  circle A12 centre (90, 290) radius 5
  circle A13 centre (10, 290) radius 5
  circle A14 centre (-70, 290) radius 5
  circle A15 centre (-30, 290) radius 5
  circle A16 centre (50, 290) radius 5
  circle A17 centre (70, 310) radius 5
  circle A18 centre (-10, 310) radius 5
  circle A19 centre (-90, 310) radius 5
  circle A20 centre (-30, 330) radius 5
  circle A21 centre (50, 330) radius 5
  circle A22 centre (70, 330) radius 5
  circle A23 centre (-10, 330) radius 5
  circle A24 centre (-90, 330) radius 5
  circle A25 centre (-30, 310) radius 5
  circle A26 centre (50, 310) radius 5
  circle A27 centre (70, 290) radius 5
  circle A28 centre (-10, 290) radius 5
  circle A29 centre (-90, 290) radius 5
  line L4 (120, 0) -> (120, 330.95)
  line L5 (120, 330.95) -> (126.35, 330.95)
  line L6 (126.35, 330.95) -> (126.35, 311.9)
  line L7 (126.35, 311.9) -> (136.5, 311.9)
  line L8 (136.5, 311.9) -> (136.5, 350)
  line L9 (136.5, 350) -> (19.05, 350)
  line L10 (19.05, 350) -> (19.05, 370)
  line L11 (19.05, 370) -> (-19.05, 370)
  line L12 (-19.05, 370) -> (-19.05, 350)
  line L13 (-19.05, 350) -> (-136.5, 350)
  line L14 (-136.5, 350) -> (-136.5, 311.9)
  line L15 (-136.5, 311.9) -> (-126.35, 311.9)
  line L16 (-126.35, 311.9) -> (-126.35, 330.95)
  line L17 (-126.35, 330.95) -> (-120, 330.95)
  line L18 (-120, 330.95) -> (-120, 0)
  line L19 (-120, 0) -> (120, 0)
  line L20 (43.7, 0) -> (107.3, 0)
  line L21 (107.3, 0) -> (107.3, 25.4)
  line L22 (107.3, 25.4) -> (43.7, 25.4)
  line L23 (43.7, 25.4) -> (43.7, 0)
  dimension "d197" = 25.4
  dimension "d198" = 12.7
  dimension "d199" = 63.6
  constraint horizontal L20
  constraint vertical L21
  constraint horizontal L22
  constraint vertical L23
  constraint coincident L19 L20.start
  measures "d197" distance of L20.start L22.end
  measures "d198" distance of L4 L21
  measures "d199" distance of L21.end L22.end
extrude "Extrude1''''" cut sketch "Sketch1 (5)" against normal blind 6.35 contours L19 L20 L21 L22 L23 bodies 5 in component "Back Wall"
sketch "Sketch2 (4)" plane through (0, 0, 356.35) normal (0, 0, 1) x (-1, 0, 0) in component "Roof"
  line L0 (19.05, -257.175) -> (19.05, -263.525)
  line L1 (19.05, -263.525) -> (-19.05, -263.525)
  line L2 (-19.05, -263.525) -> (-19.05, -257.175)
  line L3 (-19.05, -257.175) -> (19.05, -257.175)
  line L4 (-126.35, -111.125) -> (-120, -111.125)
  line L5 (-120, -111.125) -> (-120, -149.225)
  line L6 (-120, -149.225) -> (-126.35, -149.225)
  line L7 (-126.35, -149.225) -> (-126.35, -111.125)
  line L8 (-19.05, 3.075) -> (19.05, 3.075)
  line L9 (19.05, 3.075) -> (19.05, -3.275)
  line L10 (19.05, -3.275) -> (-19.05, -3.275)
  line L11 (-19.05, -3.275) -> (-19.05, 3.075)
  line L12 (120, -111.1333) -> (126.35, -111.1333)
  line L13 (126.35, -111.1333) -> (126.35, -149.2333)
  line L14 (126.35, -149.2333) -> (120, -149.2333)
  line L15 (120, -149.2333) -> (120, -111.1333)
  line L16 (136.35, 13.325) -> (-136.35, 13.325)
  line L17 (-136.35, 13.325) -> (-136.35, -273.775)
  line L18 (-136.35, -273.775) -> (136.35, -273.775)
  line L19 (136.35, -273.775) -> (136.35, 13.325)
  circle A0 centre (0, -130.225) radius 14.5
  dimension "d206" = 143.55
  dimension "d207" = 287.1
  dimension "d208" = 29
  measures "d206" distance of L18 A0.centre
  measures "d207" distance of L16 L18
  measures "d208" diameter of A0
extrude "Extrude2'''" cut sketch "Sketch2 (4)" against normal blind 10 contours A0 bodies 9 in component "Roof"
sketch "Sketch6 (2)" plane through (126.35, 0, 0) normal (1, 0, 0) x (0, 1, 0)
  line L0 (149.225, 31.75) -> (149.225, 25.4)
  line L1 (149.225, 25.4) -> (111.125, 25.4)
  line L2 (111.125, 25.4) -> (111.125, 31.75)
  line L3 (111.125, 31.75) -> (149.225, 31.75)
  circle A0 centre (183.675, 290) radius 5
  circle A1 centre (98.075, 290) radius 5
  circle A2 centre (33.875, 310) radius 5
  circle A3 centre (119.475, 310) radius 5
  circle A4 centre (205.075, 310) radius 5
  circle A5 centre (183.675, 330) radius 5
  circle A6 centre (98.075, 330) radius 5
  circle A7 centre (33.875, 330) radius 5
  circle A8 centre (119.475, 330) radius 5
  circle A9 centre (205.075, 330) radius 5
  circle A10 centre (183.675, 310) radius 5
  circle A11 centre (98.075, 310) radius 5
  circle A12 centre (33.875, 290) radius 5
  circle A13 centre (119.475, 290) radius 5
  circle A14 centre (205.075, 290) radius 5
  circle A15 centre (162.275, 290) radius 5
  circle A16 centre (76.675, 290) radius 5
  circle A17 centre (55.275, 310) radius 5
  circle A18 centre (162.275, 310) radius 5
  circle A19 centre (226.4722, 310.344) radius 5
  circle A20 centre (162.275, 330) radius 5
  circle A21 centre (76.675, 330) radius 5
  circle A22 centre (55.275, 330) radius 5
  circle A23 centre (140.875, 330) radius 5
  circle A24 centre (226.475, 330) radius 5
  circle A25 centre (140.875, 310) radius 5
  circle A26 centre (76.675, 310) radius 5
  circle A27 centre (55.275, 290) radius 5
  circle A28 centre (140.875, 290) radius 5
  circle A29 centre (226.475, 290) radius 5
  line L4 (3.175, 350) -> (3.175, 330.95)
  line L5 (3.175, 330.95) -> (-3.175, 330.95)
  line L6 (-3.175, 330.95) -> (-3.175, 350)
  line L7 (-3.175, 350) -> (-13.325, 350)
  line L8 (-13.325, 350) -> (-13.325, 311.9)
  line L9 (-13.325, 311.9) -> (3.175, 311.9)
  line L10 (3.175, 311.9) -> (3.175, 0)
  line L11 (3.175, 0) -> (257.175, 0)
  line L12 (257.175, 0) -> (257.175, 311.9)
  line L13 (257.175, 311.9) -> (273.675, 311.9)
  line L14 (273.675, 311.9) -> (273.675, 350)
  line L15 (273.675, 350) -> (263.525, 350)
  line L16 (263.525, 350) -> (263.525, 330.95)
  line L17 (263.525, 330.95) -> (257.175, 330.95)
  line L18 (257.175, 330.95) -> (257.175, 350)
  line L19 (257.175, 350) -> (149.225, 350)
  line L20 (149.225, 350) -> (149.225, 370)
  line L21 (149.225, 370) -> (111.125, 370)
  line L22 (111.125, 370) -> (111.125, 350)
  line L23 (111.125, 350) -> (3.175, 350)
  circle A30 centre (130.175, 177.8) radius 31.75
  dimension "d213" = 63.5
  dimension "d214" = 127
  dimension "d215" = 177.8
  measures "d213" diameter of A30
  measures "d214" distance of L10 A30.centre
  measures "d215" distance of L11 A30.centre
extrude "Extrude6" cut sketch "Sketch6 (2)" against normal blind 40 contours A30 bodies 2 in component "Right wall"
sketch "Sketch7" plane through (126.35, 0, 0) normal (1, 0, 0) x (0, 1, 0)
  circle A0 centre (130.175, 177.8) radius 31.75
  line L0 (149.225, 31.75) -> (149.225, 25.4)
  line L1 (149.225, 25.4) -> (111.125, 25.4)
  line L2 (111.125, 25.4) -> (111.125, 31.75)
  line L3 (111.125, 31.75) -> (149.225, 31.75)
  circle A1 centre (183.675, 290) radius 5
  circle A2 centre (98.075, 290) radius 5
  circle A3 centre (33.875, 310) radius 5
  circle A4 centre (119.475, 310) radius 5
  circle A5 centre (205.075, 310) radius 5
  circle A6 centre (183.675, 330) radius 5
  circle A7 centre (98.075, 330) radius 5
  circle A8 centre (33.875, 330) radius 5
  circle A9 centre (119.475, 330) radius 5
  circle A10 centre (205.075, 330) radius 5
  circle A11 centre (183.675, 310) radius 5
  circle A12 centre (98.075, 310) radius 5
  circle A13 centre (33.875, 290) radius 5
  circle A14 centre (119.475, 290) radius 5
  circle A15 centre (205.075, 290) radius 5
  circle A16 centre (162.275, 290) radius 5
  circle A17 centre (76.675, 290) radius 5
  circle A18 centre (55.275, 310) radius 5
  circle A19 centre (162.275, 310) radius 5
  circle A20 centre (226.4722, 310.344) radius 5
  circle A21 centre (162.275, 330) radius 5
  circle A22 centre (76.675, 330) radius 5
  circle A23 centre (55.275, 330) radius 5
  circle A24 centre (140.875, 330) radius 5
  circle A25 centre (226.475, 330) radius 5
  circle A26 centre (140.875, 310) radius 5
  circle A27 centre (76.675, 310) radius 5
  circle A28 centre (55.275, 290) radius 5
  circle A29 centre (140.875, 290) radius 5
  circle A30 centre (226.475, 290) radius 5
  line L4 (3.175, 350) -> (3.175, 330.95)
  line L5 (3.175, 330.95) -> (-3.175, 330.95)
  line L6 (-3.175, 330.95) -> (-3.175, 350)
  line L7 (-3.175, 350) -> (-13.325, 350)
  line L8 (-13.325, 350) -> (-13.325, 311.9)
  line L9 (-13.325, 311.9) -> (3.175, 311.9)
  line L10 (3.175, 311.9) -> (3.175, 0)
  line L11 (3.175, 0) -> (257.175, 0)
  line L12 (257.175, 0) -> (257.175, 311.9)
  line L13 (257.175, 311.9) -> (273.675, 311.9)
  line L14 (273.675, 311.9) -> (273.675, 350)
  line L15 (273.675, 350) -> (263.525, 350)
  line L16 (263.525, 350) -> (263.525, 330.95)
  line L17 (263.525, 330.95) -> (257.175, 330.95)
  line L18 (257.175, 330.95) -> (257.175, 350)
  line L19 (257.175, 350) -> (149.225, 350)
  line L20 (149.225, 350) -> (149.225, 370)
  line L21 (149.225, 370) -> (111.125, 370)
  line L22 (111.125, 370) -> (111.125, 350)
  line L23 (111.125, 350) -> (3.175, 350)
sketch "Sketch1 (6)" plane through (-126.35, 0, 0) normal (-1, 0, 0) x (0, -1, 0) in component "Left Wall"
  line L0 (-149.225, 25.4) -> (-149.225, 31.75)
  line L1 (-149.225, 31.75) -> (-111.125, 31.75)
  line L2 (-111.125, 31.75) -> (-111.125, 25.4)
  line L3 (-111.125, 25.4) -> (-149.225, 25.4)
  circle A0 centre (-183.675, 290) radius 5
  circle A1 centre (-98.075, 290) radius 5
  circle A2 centre (-33.875, 310) radius 5
  circle A3 centre (-119.475, 310) radius 5
  circle A4 centre (-205.075, 310) radius 5
  circle A5 centre (-183.675, 330) radius 5
  circle A6 centre (-98.075, 330) radius 5
  circle A7 centre (-33.875, 330) radius 5
  circle A8 centre (-119.475, 330) radius 5
  circle A9 centre (-205.075, 330) radius 5
  circle A10 centre (-183.675, 310) radius 5
  circle A11 centre (-98.075, 310) radius 5
  circle A12 centre (-33.875, 290) radius 5
  circle A13 centre (-119.475, 290) radius 5
  circle A14 centre (-205.075, 290) radius 5
  circle A15 centre (-162.275, 290) radius 5
  circle A16 centre (-76.675, 290) radius 5
  circle A17 centre (-55.275, 310) radius 5
  circle A18 centre (-162.275, 310) radius 5
  circle A19 centre (-226.4722, 310.344) radius 5
  circle A20 centre (-162.275, 330) radius 5
  circle A21 centre (-76.675, 330) radius 5
  circle A22 centre (-55.275, 330) radius 5
  circle A23 centre (-140.875, 330) radius 5
  circle A24 centre (-226.475, 330) radius 5
  circle A25 centre (-140.875, 310) radius 5
  circle A26 centre (-76.675, 310) radius 5
  circle A27 centre (-55.275, 290) radius 5
  circle A28 centre (-140.875, 290) radius 5
  circle A29 centre (-226.475, 290) radius 5
  line L4 (-3.175, 330.95) -> (-3.175, 350)
  line L5 (-3.175, 350) -> (-111.125, 350)
  line L6 (-111.125, 350) -> (-111.125, 370)
  line L7 (-111.125, 370) -> (-149.225, 370)
  line L8 (-149.225, 370) -> (-149.225, 350)
  line L9 (-149.225, 350) -> (-257.175, 350)
  line L10 (-257.175, 350) -> (-257.175, 330.95)
  line L11 (-257.175, 330.95) -> (-263.525, 330.95)
  line L12 (-263.525, 330.95) -> (-263.525, 350)
  line L13 (-263.525, 350) -> (-273.675, 350)
  line L14 (-273.675, 350) -> (-273.675, 311.9)
  line L15 (-273.675, 311.9) -> (-257.175, 311.9)
  line L16 (-257.175, 311.9) -> (-257.175, 0)
  line L17 (-257.175, 0) -> (-3.175, 0)
  line L18 (-3.175, 0) -> (-3.175, 311.9)
  line L19 (-3.175, 311.9) -> (13.325, 311.9)
  line L20 (13.325, 311.9) -> (13.325, 350)
  line L21 (13.325, 350) -> (3.175, 350)
  line L22 (3.175, 350) -> (3.175, 330.95)
  line L23 (3.175, 330.95) -> (-3.175, 330.95)
  circle A30 centre (-130.175, 177.8) radius 31.75
  dimension "d219" = 63.5
  dimension "d220" = 177.8
  dimension "d221" = 127
  measures "d219" diameter of A30
  measures "d220" distance of L17 A30.centre
  measures "d221" distance of L18 A30.centre
extrude "Extrude1'''''" cut sketch "Sketch1 (6)" against normal blind 20 contours A30 bodies 6 in component "Left Wall"
sketch "Sketch8" plane through (0, 263.525, 0) normal (0, 1, 0) x (-1, 0, 0)
  line L0 (107.3, 25.4) -> (107.3, 0)
  line L1 (107.3, 0) -> (120, 0)
  line L2 (120, 0) -> (120, 330.95)
  line L3 (120, 330.95) -> (126.35, 330.95)
  line L4 (126.35, 330.95) -> (126.35, 311.9)
  line L5 (126.35, 311.9) -> (136.5, 311.9)
  line L6 (136.5, 311.9) -> (136.5, 350)
  line L7 (136.5, 350) -> (19.05, 350)
  line L8 (19.05, 350) -> (19.05, 370)
  line L9 (19.05, 370) -> (-19.05, 370)
  line L10 (-19.05, 370) -> (-19.05, 350)
  line L11 (-19.05, 350) -> (-136.5, 350)
  line L12 (-136.5, 350) -> (-136.5, 311.9)
  line L13 (-136.5, 311.9) -> (-126.35, 311.9)
  line L14 (-126.35, 311.9) -> (-126.35, 330.95)
  line L15 (-126.35, 330.95) -> (-120, 330.95)
  line L16 (-120, 330.95) -> (-120, 0)
  line L17 (-120, 0) -> (43.7, 0)
  line L18 (43.7, 0) -> (43.7, 25.4)
  line L19 (43.7, 25.4) -> (107.3, 25.4)
  line L20 (-19.05, 25.4) -> (-19.05, 31.75)
  line L21 (-19.05, 31.75) -> (19.05, 31.75)
  line L22 (19.05, 31.75) -> (19.05, 25.4)
  line L23 (19.05, 25.4) -> (-19.05, 25.4)
  circle A0 centre (-50, 290) radius 5
  circle A1 centre (30, 290) radius 5
  circle A2 centre (90, 310) radius 5
  circle A3 centre (10, 310) radius 5
  circle A4 centre (-70, 310) radius 5
  circle A5 centre (-50, 330) radius 5
  circle A6 centre (30, 330) radius 5
  circle A7 centre (90, 330) radius 5
  circle A8 centre (10, 330) radius 5
  circle A9 centre (-70, 330) radius 5
  circle A10 centre (-50, 310) radius 5
  circle A11 centre (30, 310) radius 5
  circle A12 centre (90, 290) radius 5
  circle A13 centre (10, 290) radius 5
  circle A14 centre (-70, 290) radius 5
  circle A15 centre (-30, 290) radius 5
  circle A16 centre (50, 290) radius 5
  circle A17 centre (70, 310) radius 5
  circle A18 centre (-10, 310) radius 5
  circle A19 centre (-90, 310) radius 5
  circle A20 centre (-30, 330) radius 5
  circle A21 centre (50, 330) radius 5
  circle A22 centre (70, 330) radius 5
  circle A23 centre (-10, 330) radius 5
  circle A24 centre (-90, 330) radius 5
  circle A25 centre (-30, 310) radius 5
  circle A26 centre (50, 310) radius 5
  circle A27 centre (70, 290) radius 5
  circle A28 centre (-10, 290) radius 5
  circle A29 centre (-90, 290) radius 5
  line L24 (-10, 55.75) -> (10, 55.75)
  line L25 (10, 55.75) -> (10, 43.75)
  line L26 (10, 43.75) -> (-10, 43.75)
  line L27 (-10, 43.75) -> (-10, 55.75)
  line L28 (20, 55.75) -> (40, 55.75)
  line L29 (40, 55.75) -> (40, 43.75)
  line L30 (40, 43.75) -> (20, 43.75)
  line L31 (20, 43.75) -> (20, 55.75)
  line L32 (-20, 55.75) -> (-40, 55.75)
  line L33 (-40, 55.75) -> (-40, 43.75)
  line L34 (-40, 43.75) -> (-20, 43.75)
  line L35 (-20, 43.75) -> (-20, 55.75)
  dimension "d224" = 20
  dimension "d225" = 12
  dimension "d226" = 12
  dimension "d227" = 10
  dimension "d228" = 20
  dimension "d229" = 10
  dimension "d230" = 12
  dimension "d231" = 12
  dimension "d232" = 20
  dimension "d233" = 12
  dimension "d234" = 12
  dimension "d235" = 10
  constraint horizontal L24
  constraint vertical L25
  constraint horizontal L26
  constraint vertical L27
  constraint horizontal L28
  constraint vertical L29
  constraint horizontal L30
  constraint vertical L31
  constraint horizontal L32
  constraint vertical L33
  constraint horizontal L34
  constraint vertical L35
  measures "d224" distance of L24.start L24.end
  measures "d225" distance of L24.start L26.end
  measures "d226" distance of L21 L26
  measures "d227" distance of origin L27
  measures "d228" distance of L28.start L28.end
  measures "d229" distance of L25 L31
  measures "d230" distance of L28.end L29.end
  measures "d231" distance of L21 L30
  measures "d232" distance of L32.start L32.end
  measures "d233" distance of L32.end L33.end
  measures "d234" distance of L21 L34
  measures "d235" distance of L27 L35
extrude "Extrude2''''" cut sketch "Sketch8" against normal blind 15 contours L24 L25 L26 L27 | L28 L29 L30 L31 | L32 L33 L34 L35 bodies 5 in component "Back Wall"